Autodesk Fusion 360 part; units mm, degrees
(part 2 of 5)
  line L948 (107.395, 88.0223) -> (106.594, 88.0223)
  line L949 (102.344, 88.0223) -> (102.344, 93.8223)
  line L950 (121.394, 96.9215) -> (121.394, 97.9219)
  line L951 (50.2447, 93.8223) -> (50.2447, 88.0223)
  line L952 (107.395, 96.9215) -> (106.594, 96.9215)
  line L953 (68.4939, 93.8223) -> (69.2947, 93.8223)
  line L954 (87.5439, 96.9215) -> (87.5439, 93.8223)
  line L955 (88.3447, 96.9215) -> (87.5439, 96.9215)
  line L956 (35.669, 93.8223) -> (36.4698, 93.8223)
  line L957 (2.6197, 97.9219) -> (2.6197, 96.9215)
  line L958 (2.6197, 96.9215) -> (1.819, 96.9215)
  line L959 (21.6697, 93.8223) -> (21.6697, 88.0223)
  line L960 (50.2447, 97.9219) -> (50.2447, 96.9215)
  line L961 (88.3447, 83.9227) -> (102.344, 83.9227)
  line L962 (2.6197, 93.8223) -> (2.6197, 88.0223)
  line L963 (2.6197, 88.0223) -> (1.819, 88.0223)
  line L964 (2.6197, 83.9227) -> (16.6192, 83.9227)
  line L965 (88.3447, 84.9217) -> (88.3447, 83.9227)
  line L966 (121.394, 84.9217) -> (122.195, 84.9217)
  line L967 (103.145, 93.8223) -> (103.145, 96.9215)
  line L968 (88.3447, 88.0223) -> (87.5439, 88.0223)
  line L969 (102.344, 97.9219) -> (88.3447, 97.9219)
  line L970 (84.0948, 96.9215) -> (83.294, 96.9215)
  line L971 (87.5439, 88.0223) -> (87.5439, 84.9217)
  line L972 (102.344, 96.9215) -> (102.344, 97.9219)
  line L973 (122.195, 96.9215) -> (121.394, 96.9215)
  line L974 (121.394, 88.0223) -> (121.394, 93.8223)
  line L975 (103.145, 84.9217) -> (103.145, 88.0223)
  line L976 (122.195, 84.9217) -> (122.195, 88.0223)
  line L977 (83.294, 96.9215) -> (83.294, 97.9219)
  line L978 (84.0948, 84.9217) -> (84.0948, 88.0223)
  line L979 (87.5439, 84.9217) -> (88.3447, 84.9217)
  line L980 (87.5439, 93.8223) -> (88.3447, 93.8223)
  line L981 (83.294, 83.9227) -> (83.294, 84.9217)
  line L982 (83.294, 88.0223) -> (83.294, 93.8223)
  line L983 (102.344, 83.9227) -> (102.344, 84.9217)
  line L984 (83.294, 93.8223) -> (84.0948, 93.8223)
  line L985 (107.395, 84.9217) -> (107.395, 83.9227)
  line L986 (102.344, 84.9217) -> (103.145, 84.9217)
  line L987 (84.0948, 93.8223) -> (84.0948, 96.9215)
  line L988 (344.719, 12.8598) -> (345.52, 12.8598)
  line L989 (326.47, 16.9595) -> (326.47, 15.9604)
  line L990 (340.469, 16.9595) -> (326.47, 16.9595)
  line L991 (321.419, 7.0597) -> (321.419, 12.8598)
  line L992 (306.619, 12.8598) -> (307.42, 12.8598)
  line L993 (322.22, 12.8598) -> (322.22, 15.9604)
  line L994 (321.419, 16.9595) -> (307.42, 16.9595)
  line L995 (307.42, 7.0597) -> (306.619, 7.0597)
  line L996 (306.619, 7.0597) -> (306.619, 3.9605)
  line L997 (322.22, 3.9605) -> (322.22, 7.0597)
  line L998 (321.419, 12.8598) -> (322.22, 12.8598)
  line L999 (321.419, 15.9604) -> (321.419, 16.9595)
  line L1000 (306.619, 3.9605) -> (307.42, 3.9605)
  line L1001 (322.22, 15.9604) -> (321.419, 15.9604)
  line L1002 (133.587, 17.6237) -> (133.587, 17.0215)
  line L1003 (307.42, 15.9604) -> (306.619, 15.9604)
  line L1004 (307.42, 12.8598) -> (307.42, 7.0597)
  line L1005 (307.42, 3.9605) -> (307.42, 2.96)
  line L1006 (322.22, 7.0597) -> (321.419, 7.0597)
  line L1007 (307.42, 16.9595) -> (307.42, 15.9604)
  line L1008 (306.619, 15.9604) -> (306.619, 12.8598)
  line L1009 (321.419, 2.96) -> (321.419, 3.9605)
  line L1010 (307.42, 2.96) -> (321.419, 2.96)
  line L1011 (321.419, 3.9605) -> (322.22, 3.9605)
  line L1012 (340.469, 15.9604) -> (340.469, 16.9595)
  line L1013 (132.063, 7.9527) -> (132.063, 12.423)
  line L1014 (166.926, 12.423) -> (166.926, 11.8222)
  line L1015 (133.587, 20.7216) -> (132.788, 20.7216)
  line L1016 (185.688, 11.8222) -> (185.688, 12.423)
  line L1017 (133.587, 21.722) -> (133.587, 20.7216)
  line L1018 (185.688, 7.7225) -> (185.688, 8.7216)
  line L1019 (147.588, 8.7216) -> (148.387, 8.7216)
  line L1020 (186.487, 8.7216) -> (186.487, 11.8222)
  line L1021 (133.587, 8.7216) -> (133.587, 7.7225)
  line L1022 (122.276, 6.7524) -> (125.575, 6.7524)
  line L1023 (133.587, 7.7225) -> (147.588, 7.7225)
  line L1024 (132.788, 20.7216) -> (132.788, 17.6237)
  line L1025 (132.788, 17.6237) -> (133.587, 17.6237)
  line L1026 (219.826, 8.7216) -> (219.826, 11.8222)
  line L1027 (205.026, 7.7225) -> (219.025, 7.7225)
  line L1028 (166.125, 8.7216) -> (166.926, 8.7216)
  line L1029 (205.026, 12.423) -> (205.026, 11.8222)
  line L1030 (219.025, 11.8222) -> (219.025, 12.423)
  line L1031 (185.688, 8.7216) -> (186.487, 8.7216)
  line L1032 (166.926, 11.8222) -> (166.125, 11.8222)
  line L1033 (133.587, 11.8222) -> (132.788, 11.8222)
  line L1034 (147.588, 7.7225) -> (147.588, 8.7216)
  line L1035 (219.025, 8.7216) -> (219.826, 8.7216)
  line L1036 (166.926, 8.7216) -> (166.926, 7.7225)
  line L1037 (219.826, 11.8222) -> (219.025, 11.8222)
  line L1038 (148.387, 11.8222) -> (147.588, 11.8222)
  line L1039 (205.026, 21.722) -> (205.026, 20.7216)
  line L1040 (185.688, 17.0215) -> (185.688, 17.6237)
  line L1041 (147.588, 20.7216) -> (147.588, 21.722)
  line L1042 (219.025, 17.0215) -> (219.025, 17.6237)
  line L1043 (132.788, 8.7216) -> (133.587, 8.7216)
  line L1044 (205.026, 8.7216) -> (205.026, 7.7225)
  line L1045 (219.025, 7.7225) -> (219.025, 8.7216)
  line L1046 (133.587, 12.423) -> (133.587, 11.8222)
  line L1047 (196.751, 12.423) -> (196.751, 7.9527)
  line L1048 (132.788, 11.8222) -> (132.788, 8.7216)
  line L1049 (148.387, 8.7216) -> (148.387, 11.8222)
  line L1050 (166.926, 7.7225) -> (185.688, 7.7225)
  line L1051 (203.501, 17.0215) -> (203.501, 19.2517)
  line L1052 (186.487, 11.8222) -> (185.688, 11.8222)
  line L1053 (204.225, 17.6237) -> (205.026, 17.6237)
  line L1054 (202.501, 20.2517) -> (197.751, 20.2517)
  line L1055 (186.487, 20.7216) -> (185.688, 20.7216)
  line L1056 (166.125, 17.6237) -> (166.926, 17.6237)
  line L1057 (204.225, 11.8222) -> (204.225, 8.7216)
  line L1058 (205.026, 11.8222) -> (204.225, 11.8222)
  line L1059 (166.125, 11.8222) -> (166.125, 8.7216)
  line L1060 (219.025, 17.6237) -> (219.826, 17.6237)
  line L1061 (204.225, 8.7216) -> (205.026, 8.7216)
  line L1062 (147.588, 11.8222) -> (147.588, 12.423)
  line L1063 (219.025, 21.722) -> (205.026, 21.722)
  line L1064 (148.387, 20.7216) -> (147.588, 20.7216)
  line L1065 (281.226, 17.6237) -> (281.226, 11.8222)
  line L1066 (281.226, 11.8222) -> (280.425, 11.8222)
  line L1067 (296.026, 8.7216) -> (296.026, 11.8222)
  line L1068 (219.025, 20.7216) -> (219.025, 21.722)
  line L1069 (204.225, 20.7216) -> (204.225, 17.6237)
  line L1070 (280.425, 11.8222) -> (280.425, 8.7216)
  line L1071 (186.487, 17.6237) -> (186.487, 20.7216)
  line L1072 (280.425, 8.7216) -> (281.226, 8.7216)
  line L1073 (281.226, 21.722) -> (281.226, 20.7216)
  line L1074 (166.926, 21.722) -> (166.926, 20.7216)
  line L1075 (205.026, 17.6237) -> (205.026, 17.0215)
  line L1076 (185.688, 21.722) -> (166.926, 21.722)
  line L1077 (185.688, 20.7216) -> (185.688, 21.722)
  line L1078 (185.688, 17.6237) -> (186.487, 17.6237)
  line L1079 (280.425, 17.6237) -> (281.226, 17.6237)
  line L1080 (295.225, 17.6237) -> (296.026, 17.6237)
  line L1081 (281.226, 20.7216) -> (280.425, 20.7216)
  line L1082 (148.387, 17.6237) -> (148.387, 20.7216)
  line L1083 (295.225, 8.7216) -> (296.026, 8.7216)
  line L1084 (295.225, 20.7216) -> (295.225, 21.722)
  line L1085 (154.863, 20.2517) -> (150.112, 20.2517)
  line L1086 (296.026, 17.6237) -> (296.026, 20.7216)
  line L1087 (296.026, 11.8222) -> (295.225, 11.8222)
  line L1088 (219.826, 17.6237) -> (219.826, 20.7216)
  line L1089 (238.362, 21.722) -> (238.362, 20.7216)
  line L1090 (281.226, 7.7225) -> (295.225, 7.7225)
  line L1091 (166.926, 20.7216) -> (166.125, 20.7216)
  line L1092 (296.026, 20.7216) -> (295.225, 20.7216)
  line L1093 (147.588, 17.6237) -> (148.387, 17.6237)
  line L1094 (205.026, 20.7216) -> (204.225, 20.7216)
  line L1095 (166.926, 17.6237) -> (166.926, 17.0215)
  line L1096 (295.225, 21.722) -> (281.226, 21.722)
  line L1097 (147.588, 21.722) -> (133.587, 21.722)
  line L1098 (166.125, 20.7216) -> (166.125, 17.6237)
  line L1099 (280.425, 20.7216) -> (280.425, 17.6237)
  line L1100 (281.226, 8.7216) -> (281.226, 7.7225)
  line L1101 (237.563, 20.7216) -> (237.563, 17.6237)
  line L1102 (295.225, 7.7225) -> (295.225, 8.7216)
  line L1103 (147.588, 17.0215) -> (147.588, 17.6237)
  line L1104 (238.362, 20.7216) -> (237.563, 20.7216)
  line L1105 (95.4871, 11.8222) -> (94.6877, 11.8222)
  line L1106 (21.6697, 17.6237) -> (21.6697, 11.8222)
  line L1107 (21.6697, 20.7216) -> (20.869, 20.7216)
  line L1108 (67.4261, 11.8222) -> (66.6253, 11.8222)
  line L1109 (95.4871, 17.6237) -> (95.4871, 11.8222)
  line L1110 (52.626, 21.722) -> (52.626, 20.7216)
  line L1111 (295.225, 11.8222) -> (295.225, 17.6237)
  line L1112 (237.563, 17.6237) -> (238.362, 17.6237)
  line L1113 (238.362, 7.7225) -> (252.361, 7.7225)
  line L1114 (252.361, 7.7225) -> (252.361, 8.7216)
  line L1115 (238.362, 8.7216) -> (238.362, 7.7225)
  line L1116 (20.869, 17.6237) -> (21.6697, 17.6237)
  line L1117 (66.6253, 8.7216) -> (67.4261, 8.7216)
  line L1118 (219.826, 20.7216) -> (219.025, 20.7216)
  line L1119 (237.563, 8.7216) -> (238.362, 8.7216)
  line L1120 (252.361, 11.8222) -> (252.361, 17.6237)
  line L1121 (51.8252, 11.8222) -> (51.8252, 8.7216)
  line L1122 (51.8252, 8.7216) -> (52.626, 8.7216)
  line L1123 (94.6877, 20.7216) -> (94.6877, 17.6237)
  line L1124 (20.869, 20.7216) -> (20.869, 17.6237)
  line L1125 (238.362, 11.8222) -> (237.563, 11.8222)
  line L1126 (20.869, 11.8222) -> (20.869, 8.7216)
  line L1127 (20.869, 8.7216) -> (21.6697, 8.7216)
  line L1128 (253.162, 17.6237) -> (253.162, 20.7216)
  line L1129 (95.4871, 8.7216) -> (95.4871, 7.7225)
  line L1130 (66.6253, 11.8222) -> (66.6253, 17.6237)
  line L1131 (52.626, 17.6237) -> (52.626, 11.8222)
  line L1132 (252.361, 8.7216) -> (253.162, 8.7216)
  line L1133 (21.6697, 11.8222) -> (20.869, 11.8222)
  line L1134 (110.287, 17.6237) -> (110.287, 20.7216)
  line L1135 (52.626, 11.8222) -> (51.8252, 11.8222)
  line L1136 (21.6697, 21.722) -> (21.6697, 20.7216)
  line L1137 (252.361, 21.722) -> (238.362, 21.722)
  line L1138 (252.361, 20.7216) -> (252.361, 21.722)
  line L1139 (51.8252, 17.6237) -> (52.626, 17.6237)
  line L1140 (94.6877, 8.7216) -> (95.4871, 8.7216)
  line L1141 (66.6253, 17.6237) -> (67.4261, 17.6237)
  line L1142 (52.626, 7.7225) -> (66.6253, 7.7225)
  line L1143 (253.162, 20.7216) -> (252.361, 20.7216)
  line L1144 (109.488, 7.7225) -> (109.488, 8.7216)
  line L1145 (67.4261, 20.7216) -> (66.6253, 20.7216)
  line L1146 (95.4871, 21.722) -> (95.4871, 20.7216)
  line L1147 (110.287, 11.8222) -> (109.488, 11.8222)
  line L1148 (109.488, 11.8222) -> (109.488, 17.6237)
  line L1149 (252.361, 17.6237) -> (253.162, 17.6237)
  line L1150 (253.162, 8.7216) -> (253.162, 11.8222)
  line L1151 (109.488, 21.722) -> (95.4871, 21.722)
  line L1152 (52.626, 8.7216) -> (52.626, 7.7225)
  line L1153 (95.4871, 20.7216) -> (94.6877, 20.7216)
  line L1154 (94.6877, 17.6237) -> (95.4871, 17.6237)
  line L1155 (253.162, 11.8222) -> (252.361, 11.8222)
  line L1156 (109.488, 8.7216) -> (110.287, 8.7216)
  line L1157 (206.606, 27.7716) -> (207.407, 27.7716)
  line L1158 (202.357, 36.6737) -> (203.156, 36.6737)
  line L1159 (149.456, 30.8722) -> (149.456, 27.7716)
  line L1160 (164.257, 30.8722) -> (164.257, 36.6737)
  line L1161 (221.407, 26.7725) -> (221.407, 27.7716)
  line L1162 (187.556, 39.7715) -> (187.556, 36.6737)
  line L1163 (150.257, 26.7725) -> (164.257, 26.7725)
  line L1164 (187.556, 27.7716) -> (188.357, 27.7716)
  line L1165 (202.357, 27.7716) -> (203.156, 27.7716)
  line L1166 (222.206, 30.8722) -> (221.407, 30.8722)
  line L1167 (168.506, 30.8722) -> (168.506, 27.7716)
  line L1168 (168.506, 27.7716) -> (169.307, 27.7716)
  line L1169 (183.307, 26.7725) -> (183.307, 27.7716)
  line L1170 (184.106, 39.7715) -> (183.307, 39.7715)
  line L1171 (203.156, 39.7715) -> (202.357, 39.7715)
  line L1172 (183.307, 39.7715) -> (183.307, 40.7719)
  line L1173 (188.357, 26.7725) -> (202.357, 26.7725)
  line L1174 (165.056, 36.6737) -> (165.056, 39.7715)
  line L1175 (221.407, 36.6737) -> (222.206, 36.6737)
  line L1176 (169.307, 27.7716) -> (169.307, 26.7725)
  line L1177 (165.056, 30.8722) -> (164.257, 30.8722)
  line L1178 (169.307, 40.7719) -> (169.307, 39.7715)
  line L1179 (169.307, 30.8722) -> (168.506, 30.8722)
  line L1180 (203.156, 36.6737) -> (203.156, 39.7715)
  line L1181 (150.257, 36.6737) -> (150.257, 30.8722)
  line L1182 (221.407, 30.8722) -> (221.407, 36.6737)
  line L1183 (150.257, 27.7716) -> (150.257, 26.7725)
  line L1184 (169.307, 39.7715) -> (168.506, 39.7715)
  line L1185 (184.106, 27.7716) -> (184.106, 30.8722)
  line L1186 (203.156, 30.8722) -> (202.357, 30.8722)
  line L1187 (168.506, 39.7715) -> (168.506, 36.6737)
  line L1188 (149.456, 27.7716) -> (150.257, 27.7716)
  line L1189 (150.257, 30.8722) -> (149.456, 30.8722)
  line L1190 (164.257, 36.6737) -> (165.056, 36.6737)
  line L1191 (188.357, 39.7715) -> (187.556, 39.7715)
  line L1192 (188.357, 36.6737) -> (188.357, 30.8722)
  line L1193 (202.357, 26.7725) -> (202.357, 27.7716)
  line L1194 (203.156, 27.7716) -> (203.156, 30.8722)
  line L1195 (207.407, 26.7725) -> (221.407, 26.7725)
  line L1196 (221.407, 27.7716) -> (222.206, 27.7716)
  line L1197 (164.257, 27.7716) -> (165.056, 27.7716)
  line L1198 (169.307, 26.7725) -> (183.307, 26.7725)
  line L1199 (202.357, 30.8722) -> (202.357, 36.6737)
  line L1200 (202.357, 39.7715) -> (202.357, 40.7719)
  line L1201 (222.206, 27.7716) -> (222.206, 30.8722)
  line L1202 (150.257, 40.7719) -> (150.257, 39.7715)
  line L1203 (183.307, 36.6737) -> (184.106, 36.6737)
  line L1204 (184.106, 36.6737) -> (184.106, 39.7715)
  line L1205 (183.307, 30.8722) -> (183.307, 36.6737)
  line L1206 (169.307, 36.6737) -> (169.307, 30.8722)
  line L1207 (164.257, 26.7725) -> (164.257, 27.7716)
  line L1208 (165.056, 27.7716) -> (165.056, 30.8722)
  line L1209 (202.357, 40.7719) -> (188.357, 40.7719)
  line L1210 (360.32, 12.8598) -> (360.32, 15.9604)
  line L1211 (326.47, 15.9604) -> (325.669, 15.9604)
  line L1212 (345.52, 16.9595) -> (345.52, 15.9604)
  line L1213 (344.719, 3.9605) -> (345.52, 3.9605)
  line L1214 (325.669, 15.9604) -> (325.669, 12.8598)
  line L1215 (341.27, 15.9604) -> (340.469, 15.9604)
  line L1216 (183.307, 27.7716) -> (184.106, 27.7716)
  line L1217 (188.357, 30.8722) -> (187.556, 30.8722)
  line L1218 (150.257, 39.7715) -> (149.456, 39.7715)
  line L1219 (183.307, 40.7719) -> (169.307, 40.7719)
  line L1220 (340.469, 2.96) -> (340.469, 3.9605)
  line L1221 (326.47, 3.9605) -> (326.47, 2.96)
  line L1222 (345.52, 15.9604) -> (344.719, 15.9604)
  line L1223 (359.519, 12.8598) -> (360.32, 12.8598)
  line L1224 (341.27, 3.9605) -> (341.27, 7.0597)
  line L1225 (345.52, 7.0597) -> (344.719, 7.0597)
  line L1226 (359.519, 2.96) -> (359.519, 3.9605)
  line L1227 (360.32, 7.0597) -> (359.519, 7.0597)
  line L1228 (345.52, 3.9605) -> (345.52, 2.96)
  line L1229 (359.519, 16.9595) -> (345.52, 16.9595)
  line L1230 (325.669, 3.9605) -> (326.47, 3.9605)
  line L1231 (168.506, 36.6737) -> (169.307, 36.6737)
  line L1232 (341.27, 12.8598) -> (341.27, 15.9604)
  line L1233 (344.719, 7.0597) -> (344.719, 3.9605)
  line L1234 (360.32, 15.9604) -> (359.519, 15.9604)
  line L1235 (344.719, 15.9604) -> (344.719, 12.8598)
  line L1236 (221.407, 39.7715) -> (221.407, 40.7719)
  line L1237 (149.456, 36.6737) -> (150.257, 36.6737)
  line L1238 (345.52, 2.96) -> (359.519, 2.96)
  line L1239 (326.47, 12.8598) -> (326.47, 7.0597)
  line L1240 (187.556, 30.8722) -> (187.556, 27.7716)
  line L1241 (187.556, 36.6737) -> (188.357, 36.6737)
  line L1242 (149.456, 39.7715) -> (149.456, 36.6737)
  line L1243 (341.27, 7.0597) -> (340.469, 7.0597)
  line L1244 (359.519, 3.9605) -> (360.32, 3.9605)
  line L1245 (359.519, 15.9604) -> (359.519, 16.9595)
  line L1246 (359.519, 7.0597) -> (359.519, 12.8598)
  line L1247 (222.206, 39.7715) -> (221.407, 39.7715)
  line L1248 (184.106, 30.8722) -> (183.307, 30.8722)
  line L1249 (222.206, 36.6737) -> (222.206, 39.7715)
  line L1250 (326.47, 2.96) -> (340.469, 2.96)
  line L1251 (340.469, 3.9605) -> (341.27, 3.9605)
  line L1252 (340.469, 7.0597) -> (340.469, 12.8598)
  line L1253 (340.469, 12.8598) -> (341.27, 12.8598)
  line L1254 (360.32, 3.9605) -> (360.32, 7.0597)
  line L1255 (188.357, 27.7716) -> (188.357, 26.7725)
  line L1256 (325.669, 12.8598) -> (326.47, 12.8598)
  line L1257 (325.669, 7.0597) -> (325.669, 3.9605)
  line L1258 (207.407, 27.7716) -> (207.407, 26.7725)
  line L1259 (345.52, 12.8598) -> (345.52, 7.0597)
  line L1260 (221.407, 40.7719) -> (207.407, 40.7719)
  line L1261 (326.47, 7.0597) -> (325.669, 7.0597)
  line L1262 (188.357, 40.7719) -> (188.357, 39.7715)
  line L1263 (135.169, 74.7723) -> (135.97, 74.7723)
  line L1264 (135.97, 64.8727) -> (149.969, 64.8727)
  line L1265 (97.8697, 77.8715) -> (97.0689, 77.8715)
  line L1266 (169.019, 78.8719) -> (155.02, 78.8719)
  line L1267 (149.969, 65.8717) -> (150.77, 65.8717)
  line L1268 (97.0689, 77.8715) -> (97.0689, 74.7723)
  line L1269 (131.72, 65.8717) -> (131.72, 68.9723)
  line L1270 (116.92, 77.8715) -> (116.119, 77.8715)
  line L1271 (135.97, 68.9723) -> (135.169, 68.9723)
  line L1272 (116.92, 64.8727) -> (130.919, 64.8727)
  line L1273 (130.919, 77.8715) -> (130.919, 78.8719)
  line L1274 (116.119, 68.9723) -> (116.119, 65.8717)
  line L1275 (150.77, 74.7723) -> (150.77, 77.8715)
  line L1276 (169.019, 74.7723) -> (169.82, 74.7723)
  line L1277 (169.019, 64.8727) -> (169.019, 65.8717)
  line L1278 (131.72, 74.7723) -> (131.72, 77.8715)
  line L1279 (155.02, 68.9723) -> (154.219, 68.9723)
  line L1280 (130.919, 74.7723) -> (131.72, 74.7723)
  line L1281 (169.82, 74.7723) -> (169.82, 77.8715)
  line L1282 (149.969, 74.7723) -> (150.77, 74.7723)
  line L1283 (135.169, 77.8715) -> (135.169, 74.7723)
  line L1284 (154.219, 68.9723) -> (154.219, 65.8717)
  line L1285 (116.119, 65.8717) -> (116.92, 65.8717)
  line L1286 (131.72, 77.8715) -> (130.919, 77.8715)
  line L1287 (135.169, 68.9723) -> (135.169, 65.8717)
  line L1288 (150.77, 77.8715) -> (149.969, 77.8715)
  line L1289 (130.919, 65.8717) -> (131.72, 65.8717)
  line L1290 (135.97, 74.7723) -> (135.97, 68.9723)
  line L1291 (169.82, 68.9723) -> (169.019, 68.9723)
  line L1292 (116.92, 74.7723) -> (116.92, 68.9723)
  line L1293 (97.8697, 78.8719) -> (97.8697, 77.8715)
  line L1294 (97.0689, 74.7723) -> (97.8697, 74.7723)
  line L1295 (112.67, 74.7723) -> (112.67, 77.8715)
  line L1296 (130.919, 78.8719) -> (116.92, 78.8719)
  line L1297 (92.819, 78.8719) -> (78.8197, 78.8719)
  line L1298 (69.8059, 65.8717) -> (69.8059, 68.9723)
  line L1299 (54.2064, 65.8717) -> (55.0072, 65.8717)
  line L1300 (78.8197, 65.8717) -> (78.8197, 64.8727)
  line L1301 (55.0072, 64.8727) -> (69.0065, 64.8727)
  line L1302 (69.8059, 74.7723) -> (69.8059, 77.8715)
  line L1303 (78.8197, 68.9723) -> (78.0189, 68.9723)
  line L1304 (131.72, 68.9723) -> (130.919, 68.9723)
  line L1305 (93.6198, 77.8715) -> (92.819, 77.8715)
  line L1306 (130.919, 68.9723) -> (130.919, 74.7723)
  line L1307 (69.0065, 77.8715) -> (69.0065, 78.8719)
  line L1308 (78.0189, 65.8717) -> (78.8197, 65.8717)
  line L1309 (92.819, 65.8717) -> (93.6198, 65.8717)
  line L1310 (112.67, 65.8717) -> (112.67, 68.9723)
  line L1311 (69.0065, 64.8727) -> (69.0065, 65.8717)
  line L1312 (69.8059, 77.8715) -> (69.0065, 77.8715)
  line L1313 (69.0065, 78.8719) -> (55.0072, 78.8719)
  line L1314 (21.6697, 78.8719) -> (21.6697, 77.8715)
  line L1315 (135.97, 78.8719) -> (135.97, 77.8715)
  line L1316 (21.6697, 77.8715) -> (20.869, 77.8715)
  line L1317 (54.2064, 68.9723) -> (54.2064, 65.8717)
  line L1318 (111.869, 74.7723) -> (112.67, 74.7723)
  line L1319 (21.6697, 74.7723) -> (21.6697, 68.9723)
  line L1320 (69.0065, 74.7723) -> (69.8059, 74.7723)
  line L1321 (20.869, 77.8715) -> (20.869, 74.7723)
  line L1322 (111.869, 78.8719) -> (97.8697, 78.8719)
  line L1323 (20.869, 74.7723) -> (21.6697, 74.7723)
  line L1324 (54.2064, 77.8715) -> (54.2064, 74.7723)
  line L1325 (78.8197, 64.8727) -> (92.819, 64.8727)
  line L1326 (78.0189, 74.7723) -> (78.8197, 74.7723)
  line L1327 (97.8697, 64.8727) -> (111.869, 64.8727)
  line L1328 (78.8197, 74.7723) -> (78.8197, 68.9723)
  line L1329 (93.6198, 74.7723) -> (93.6198, 77.8715)
  line L1330 (69.8059, 68.9723) -> (69.0065, 68.9723)
  line L1331 (69.0065, 68.9723) -> (69.0065, 74.7723)
  line L1332 (78.0189, 77.8715) -> (78.0189, 74.7723)
  line L1333 (21.6697, 64.8727) -> (35.669, 64.8727)
  line L1334 (20.869, 68.9723) -> (20.869, 65.8717)
  line L1335 (92.819, 68.9723) -> (92.819, 74.7723)
  line L1336 (55.0072, 74.7723) -> (55.0072, 68.9723)
  line L1337 (111.869, 68.9723) -> (111.869, 74.7723)
  line L1338 (36.4698, 65.8717) -> (36.4698, 68.9723)
  line L1339 (93.6198, 65.8717) -> (93.6198, 68.9723)
  line L1340 (78.0189, 68.9723) -> (78.0189, 65.8717)
  line L1341 (92.819, 77.8715) -> (92.819, 78.8719)
  line L1342 (112.67, 68.9723) -> (111.869, 68.9723)
  line L1343 (35.669, 65.8717) -> (36.4698, 65.8717)
  line L1344 (92.819, 74.7723) -> (93.6198, 74.7723)
  line L1345 (21.6697, 65.8717) -> (21.6697, 64.8727)
  line L1346 (20.869, 65.8717) -> (21.6697, 65.8717)
  line L1347 (55.0072, 65.8717) -> (55.0072, 64.8727)
  line L1348 (69.0065, 65.8717) -> (69.8059, 65.8717)
  line L1349 (55.0072, 68.9723) -> (54.2064, 68.9723)
  line L1350 (35.669, 64.8727) -> (35.669, 65.8717)
  line L1351 (92.819, 64.8727) -> (92.819, 65.8717)
  line L1352 (21.6697, 68.9723) -> (20.869, 68.9723)
  line L1353 (78.8197, 77.8715) -> (78.0189, 77.8715)
  line L1354 (93.6198, 68.9723) -> (92.819, 68.9723)
  line L1355 (78.8197, 78.8719) -> (78.8197, 77.8715)
  line L1356 (112.67, 77.8715) -> (111.869, 77.8715)
  line L1357 (55.0072, 77.8715) -> (54.2064, 77.8715)
  line L1358 (54.2064, 74.7723) -> (55.0072, 74.7723)
  line L1359 (297.094, 96.9215) -> (297.094, 93.8223)
  line L1360 (304.169, 82.9525) -> (304.169, 83.9227)
  line L1361 (331.745, 88.0223) -> (330.944, 88.0223)
  line L1362 (16.6192, 78.8719) -> (2.6196, 78.8719)
  line L1363 (111.869, 77.8715) -> (111.869, 78.8719)
  line L1364 (16.6192, 64.8727) -> (16.6192, 65.8717)
  line L1365 (35.669, 77.8715) -> (35.669, 78.8719)
  line L1366 (2.6197, 74.7723) -> (2.6197, 68.9723)
  line L1367 (111.869, 64.8727) -> (111.869, 65.8717)
  line L1368 (35.669, 68.9723) -> (35.669, 74.7723)
  line L1369 (17.4198, 65.8717) -> (17.4198, 68.9723)
  line L1370 (331.745, 93.8223) -> (331.745, 96.9215)
  line L1371 (297.094, 93.8223) -> (297.895, 93.8223)
  line L1372 (330.944, 97.9219) -> (297.895, 97.9219)
  line L1373 (349.481, 96.9215) -> (349.481, 93.8223)
  line L1374 (55.0072, 78.8719) -> (55.0072, 77.8715)
  line L1375 (324.67, 82.9525) -> (327.969, 82.9525)
  line L1376 (297.895, 84.9217) -> (297.895, 83.9227)
  line L1377 (111.869, 65.8717) -> (112.67, 65.8717)
  line L1378 (350.282, 93.8223) -> (350.282, 88.0223)
  line L1379 (297.895, 97.9219) -> (297.895, 96.9215)
  line L1380 (2.6197, 77.8715) -> (1.819, 77.8715)
  line L1381 (36.4698, 68.9723) -> (35.669, 68.9723)
  line L1382 (330.944, 93.8223) -> (331.745, 93.8223)
  line L1383 (297.895, 88.0223) -> (297.094, 88.0223)
  line L1384 (297.895, 83.9227) -> (300.87, 83.9227)
  line L1385 (327.969, 82.9525) -> (327.969, 83.9227)
  line L1386 (327.969, 83.9227) -> (330.944, 83.9227)
  line L1387 (300.87, 82.9525) -> (304.169, 82.9525)
  line L1388 (2.6197, 78.8719) -> (2.6197, 77.8715)
  line L1389 (304.169, 83.9227) -> (324.67, 83.9227)
  line L1390 (278.044, 84.9217) -> (278.845, 84.9217)
  line L1391 (274.595, 88.0223) -> (273.794, 88.0223)
  line L1392 (16.6192, 65.8717) -> (17.4198, 65.8717)
  line L1393 (2.6197, 65.8717) -> (2.6197, 64.8727)
  line L1394 (17.4198, 74.7723) -> (17.4198, 77.8715)
  line L1395 (17.4198, 68.9723) -> (16.6192, 68.9723)
  line L1396 (349.481, 93.8223) -> (350.282, 93.8223)
  line L1397 (1.819, 74.7723) -> (2.6197, 74.7723)
  line L1398 (17.4198, 77.8715) -> (16.6192, 77.8715)
  line L1399 (278.044, 88.0223) -> (278.044, 84.9217)
  line L1400 (258.994, 84.9217) -> (259.795, 84.9217)
  line L1401 (297.094, 88.0223) -> (297.094, 84.9217)
  line L1402 (1.819, 68.9723) -> (1.819, 65.8717)
  line L1403 (1.819, 77.8715) -> (1.819, 74.7723)
  line L1404 (1.819, 65.8717) -> (2.6197, 65.8717)
  line L1405 (300.87, 83.9227) -> (300.87, 82.9525)
  line L1406 (330.944, 84.9217) -> (331.745, 84.9217)
  line L1407 (297.094, 84.9217) -> (297.895, 84.9217)
  line L1408 (35.669, 78.8719) -> (21.6697, 78.8719)
  line L1409 (16.6192, 77.8715) -> (16.6192, 78.8719)
  line L1410 (297.895, 96.9215) -> (297.094, 96.9215)
  line L1411 (35.669, 74.7723) -> (36.4698, 74.7723)
  line L1412 (16.6192, 74.7723) -> (17.4198, 74.7723)
  line L1413 (331.745, 96.9215) -> (330.944, 96.9215)
  line L1414 (331.745, 84.9217) -> (331.745, 88.0223)
  line L1415 (2.6197, 64.8727) -> (16.6192, 64.8727)
  line L1416 (330.944, 96.9215) -> (330.944, 97.9219)
  line L1417 (16.6192, 68.9723) -> (16.6192, 74.7723)
  line L1418 (350.282, 88.0223) -> (349.481, 88.0223)
  line L1419 (297.895, 93.8223) -> (297.895, 88.0223)
  line L1420 (36.4698, 74.7723) -> (36.4698, 77.8715)
  line L1421 (330.944, 88.0223) -> (330.944, 93.8223)
  line L1422 (349.481, 84.9217) -> (350.282, 84.9217)
  line L1423 (350.282, 84.9217) -> (350.282, 83.9227)
  line L1424 (324.67, 83.9227) -> (324.67, 82.9525)
  line L1425 (350.282, 97.9219) -> (350.282, 96.9215)
  line L1426 (350.282, 96.9215) -> (349.481, 96.9215)
  line L1427 (292.844, 93.8223) -> (293.645, 93.8223)
  line L1428 (278.845, 97.9219) -> (278.845, 96.9215)
  line L1429 (364.282, 93.8223) -> (365.083, 93.8223)
  line L1430 (292.844, 83.9227) -> (292.844, 84.9217)
  line L1431 (273.794, 84.9217) -> (274.595, 84.9217)
  line L1432 (365.083, 96.9215) -> (364.282, 96.9215)
  line L1433 (36.4698, 77.8715) -> (35.669, 77.8715)
  line L1434 (330.944, 83.9227) -> (330.944, 84.9217)
  line L1435 (364.282, 96.9215) -> (364.282, 97.9219)
  line L1436 (2.6197, 68.9723) -> (1.819, 68.9723)
  line L1437 (349.481, 88.0223) -> (349.481, 84.9217)
  line L1438 (258.994, 88.0223) -> (258.994, 84.9217)
  line L1439 (364.282, 88.0223) -> (364.282, 93.8223)
  line L1440 (240.745, 97.9219) -> (240.745, 96.9215)
  line L1441 (240.745, 96.9215) -> (239.944, 96.9215)
  line L1442 (239.944, 93.8223) -> (240.745, 93.8223)
  line L1443 (240.745, 93.8223) -> (240.745, 88.0223)
  line L1444 (240.745, 88.0223) -> (239.944, 88.0223)
  line L1445 (278.044, 93.8223) -> (278.845, 93.8223)
  line L1446 (274.595, 93.8223) -> (274.595, 96.9215)
  line L1447 (273.794, 93.8223) -> (274.595, 93.8223)
  line L1448 (239.944, 84.9217) -> (240.745, 84.9217)
  line L1449 (240.745, 83.9227) -> (254.744, 83.9227)
  line L1450 (254.744, 83.9227) -> (254.744, 84.9217)
  line L1451 (365.083, 88.0223) -> (364.282, 88.0223)
  line L1452 (273.794, 83.9227) -> (273.794, 84.9217)
  line L1453 (364.282, 97.9219) -> (350.282, 97.9219)
  line L1454 (278.845, 96.9215) -> (278.044, 96.9215)
  line L1455 (365.083, 93.8223) -> (365.083, 96.9215)
  line L1456 (240.745, 84.9217) -> (240.745, 83.9227)
  line L1457 (255.545, 84.9217) -> (255.545, 88.0223)
  line L1458 (278.845, 88.0223) -> (278.044, 88.0223)
  line L1459 (292.844, 97.9219) -> (278.845, 97.9219)
  line L1460 (254.744, 84.9217) -> (255.545, 84.9217)
  line L1461 (274.595, 96.9215) -> (273.794, 96.9215)
  line L1462 (292.844, 96.9215) -> (292.844, 97.9219)
  line L1463 (259.795, 88.0223) -> (258.994, 88.0223)
  line L1464 (239.944, 96.9215) -> (239.944, 93.8223)
  line L1465 (239.944, 88.0223) -> (239.944, 84.9217)
  line L1466 (278.845, 93.8223) -> (278.845, 88.0223)
  line L1467 (273.794, 88.0223) -> (273.794, 93.8223)
  line L1468 (292.844, 84.9217) -> (293.645, 84.9217)
  line L1469 (273.794, 97.9219) -> (259.795, 97.9219)
  line L1470 (259.795, 93.8223) -> (259.795, 88.0223)
  line L1471 (292.844, 88.0223) -> (292.844, 93.8223)
  line L1472 (259.795, 96.9215) -> (258.994, 96.9215)
  line L1473 (293.645, 88.0223) -> (292.844, 88.0223)
  line L1474 (364.282, 84.9217) -> (365.083, 84.9217)
  line L1475 (293.645, 96.9215) -> (292.844, 96.9215)
  line L1476 (278.845, 84.9217) -> (278.845, 83.9227)
  line L1477 (235.694, 97.9219) -> (221.695, 97.9219)
  line L1478 (202.645, 97.9219) -> (202.645, 96.9215)
  line L1479 (183.595, 96.9215) -> (182.794, 96.9215)
  line L1480 (182.794, 96.9215) -> (182.794, 93.8223)
  line L1481 (183.595, 93.8223) -> (183.595, 88.0223)
  line L1482 (201.844, 93.8223) -> (202.645, 93.8223)
  line L1483 (235.694, 84.9217) -> (236.495, 84.9217)
  line L1484 (350.282, 83.9227) -> (364.282, 83.9227)
  line L1485 (182.794, 88.0223) -> (182.794, 84.9217)
  line L1486 (198.395, 84.9217) -> (198.395, 88.0223)
  line L1487 (197.594, 88.0223) -> (197.594, 93.8223)
  line L1488 (273.794, 96.9215) -> (273.794, 97.9219)
  line L1489 (197.594, 84.9217) -> (198.395, 84.9217)
  line L1490 (182.794, 84.9217) -> (183.595, 84.9217)
  line L1491 (258.994, 93.8223) -> (259.795, 93.8223)
  line L1492 (293.645, 84.9217) -> (293.645, 88.0223)
  line L1493 (236.495, 88.0223) -> (235.694, 88.0223)
  line L1494 (216.644, 96.9215) -> (216.644, 97.9219)
  line L1495 (183.595, 83.9227) -> (197.594, 83.9227)
  line L1496 (197.594, 83.9227) -> (197.594, 84.9217)
  line L1497 (255.545, 96.9215) -> (254.744, 96.9215)
  line L1498 (236.495, 96.9215) -> (235.694, 96.9215)
  line L1499 (216.644, 84.9217) -> (217.445, 84.9217)
  line L1500 (216.644, 97.9219) -> (202.645, 97.9219)
  line L1501 (259.795, 97.9219) -> (259.795, 96.9215)
  line L1502 (183.595, 84.9217) -> (183.595, 83.9227)
  line L1503 (202.645, 83.9227) -> (216.644, 83.9227)
  line L1504 (198.395, 88.0223) -> (197.594, 88.0223)
  line L1505 (259.795, 84.9217) -> (259.795, 83.9227)
  line L1506 (221.695, 96.9215) -> (220.894, 96.9215)
  line L1507 (220.894, 93.8223) -> (221.695, 93.8223)
  line L1508 (278.845, 83.9227) -> (292.844, 83.9227)
  line L1509 (293.645, 93.8223) -> (293.645, 96.9215)
  line L1510 (236.495, 84.9217) -> (236.495, 88.0223)
  line L1511 (254.744, 96.9215) -> (254.744, 97.9219)
  line L1512 (255.545, 93.8223) -> (255.545, 96.9215)
  line L1513 (259.795, 83.9227) -> (273.794, 83.9227)
  line L1514 (365.083, 84.9217) -> (365.083, 88.0223)
  line L1515 (274.595, 84.9217) -> (274.595, 88.0223)
  line L1516 (364.282, 83.9227) -> (364.282, 84.9217)
  line L1517 (278.044, 96.9215) -> (278.044, 93.8223)
  line L1518 (258.994, 96.9215) -> (258.994, 93.8223)
  line L1519 (201.844, 84.9217) -> (202.645, 84.9217)
  line L1520 (217.445, 93.8223) -> (217.445, 96.9215)
  line L1521 (221.695, 84.9217) -> (221.695, 83.9227)
  line L1522 (220.894, 96.9215) -> (220.894, 93.8223)
  line L1523 (202.645, 84.9217) -> (202.645, 83.9227)
  line L1524 (235.694, 83.9227) -> (235.694, 84.9217)
  line L1525 (254.744, 93.8223) -> (255.545, 93.8223)
  line L1526 (221.695, 88.0223) -> (220.894, 88.0223)
  line L1527 (236.495, 93.8223) -> (236.495, 96.9215)
  line L1528 (217.445, 88.0223) -> (216.644, 88.0223)
  line L1529 (254.744, 88.0223) -> (254.744, 93.8223)
  line L1530 (183.595, 88.0223) -> (182.794, 88.0223)
  line L1531 (197.594, 97.9219) -> (183.595, 97.9219)
  line L1532 (164.545, 93.8223) -> (164.545, 88.0223)
  line L1533 (216.644, 88.0223) -> (216.644, 93.8223)
  line L1534 (144.694, 88.0223) -> (144.694, 84.9217)
  line L1535 (255.545, 88.0223) -> (254.744, 88.0223)
  line L1536 (183.595, 97.9219) -> (183.595, 96.9215)
  line L1537 (235.694, 96.9215) -> (235.694, 97.9219)
  line L1538 (197.594, 93.8223) -> (198.395, 93.8223)
  line L1539 (235.694, 88.0223) -> (235.694, 93.8223)
  line L1540 (220.894, 88.0223) -> (220.894, 84.9217)
  line L1541 (216.644, 83.9227) -> (216.644, 84.9217)
  line L1542 (201.844, 88.0223) -> (201.844, 84.9217)
  line L1543 (221.695, 97.9219) -> (221.695, 96.9215)
  line L1544 (254.744, 97.9219) -> (240.745, 97.9219)
  line L1545 (217.445, 96.9215) -> (216.644, 96.9215)
  line L1546 (202.645, 96.9215) -> (201.844, 96.9215)
  line L1547 (198.395, 93.8223) -> (198.395, 96.9215)
  line L1548 (202.645, 88.0223) -> (201.844, 88.0223)
  line L1549 (221.695, 83.9227) -> (235.694, 83.9227)
  line L1550 (221.695, 93.8223) -> (221.695, 88.0223)
  line L1551 (235.694, 93.8223) -> (236.495, 93.8223)
  line L1552 (220.894, 84.9217) -> (221.695, 84.9217)
  line L1553 (202.645, 93.8223) -> (202.645, 88.0223)
  line L1554 (217.445, 84.9217) -> (217.445, 88.0223)
  line L1555 (216.644, 93.8223) -> (217.445, 93.8223)
  line L1556 (201.844, 96.9215) -> (201.844, 93.8223)
  line L1557 (182.794, 93.8223) -> (183.595, 93.8223)
  line L1558 (173.269, 77.8715) -> (173.269, 74.7723)
  line L1559 (169.019, 77.8715) -> (169.019, 78.8719)
  line L1560 (226.169, 68.9723) -> (226.169, 74.7723)
  line L1561 (226.169, 65.8717) -> (226.97, 65.8717)
  line L1562 (174.07, 77.8715) -> (173.269, 77.8715)
  line L1563 (97.8697, 74.7723) -> (97.8697, 68.9723)
  line L1564 (212.17, 64.8727) -> (226.169, 64.8727)
  line L1565 (207.92, 77.8715) -> (207.119, 77.8715)
  line L1566 (207.119, 78.8719) -> (193.12, 78.8719)
  line L1567 (97.8697, 68.9723) -> (97.0689, 68.9723)
  line L1568 (207.119, 64.8727) -> (207.119, 65.8717)
  line L1569 (211.369, 68.9723) -> (211.369, 65.8717)
  line L1570 (212.17, 65.8717) -> (212.17, 64.8727)
  line L1571 (174.07, 78.8719) -> (174.07, 77.8715)
  line L1572 (149.969, 68.9723) -> (149.969, 74.7723)
  line L1573 (212.17, 77.8715) -> (211.369, 77.8715)
  line L1574 (97.0689, 68.9723) -> (97.0689, 65.8717)
  line L1575 (97.0689, 65.8717) -> (97.8697, 65.8717)
  line L1576 (155.02, 64.8727) -> (169.019, 64.8727)
  line L1577 (135.169, 65.8717) -> (135.97, 65.8717)
  line L1578 (150.77, 68.9723) -> (149.969, 68.9723)
  line L1579 (116.119, 74.7723) -> (116.92, 74.7723)
  line L1580 (149.969, 77.8715) -> (149.969, 78.8719)
  line L1581 (169.82, 65.8717) -> (169.82, 68.9723)
  line L1582 (135.97, 65.8717) -> (135.97, 64.8727)
  line L1583 (169.019, 65.8717) -> (169.82, 65.8717)
  line L1584 (116.119, 77.8715) -> (116.119, 74.7723)
  line L1585 (97.8697, 65.8717) -> (97.8697, 64.8727)
  line L1586 (149.969, 64.8727) -> (149.969, 65.8717)
  line L1587 (169.82, 77.8715) -> (169.019, 77.8715)
  line L1588 (155.02, 65.8717) -> (155.02, 64.8727)
  line L1589 (135.97, 77.8715) -> (135.169, 77.8715)
  line L1590 (154.219, 65.8717) -> (155.02, 65.8717)
  line L1591 (149.969, 78.8719) -> (135.97, 78.8719)
  line L1592 (150.77, 65.8717) -> (150.77, 68.9723)
  line L1593 (169.019, 68.9723) -> (169.019, 74.7723)
  line L1594 (116.92, 78.8719) -> (116.92, 77.8715)
  line L1595 (116.92, 68.9723) -> (116.119, 68.9723)
  line L1596 (116.92, 65.8717) -> (116.92, 64.8727)
  line L1597 (130.919, 64.8727) -> (130.919, 65.8717)
  line L1598 (54.0504, 39.3016) -> (59.6225, 39.3016)
  line L1599 (60.6225, 38.3016) -> (60.6225, 26.8024)
  line L1600 (59.6225, 25.8024) -> (54.0504, 25.8024)
  line L1601 (53.0504, 26.8024) -> (53.0504, 38.3016)
  line L1602 (84.2847, 25.8024) -> (78.676, 25.8024)
  line L1603 (77.676, 26.8024) -> (77.676, 27.0027)
  line L1604 (85.2847, 38.3016) -> (85.2847, 26.8024)
  line L1605 (122.276, 6.7524) -> (120.725, 6.7524)
  line L1606 (154.863, 6.7524) -> (150.112, 6.7524)
  line L1607 (149.112, 7.7524) -> (149.112, 19.2517)
  line L1608 (202.501, 6.7524) -> (197.751, 6.7524)
  line L1609 (227.126, 6.7524) -> (221.551, 6.7524)
  line L1610 (221.551, 20.2517) -> (227.126, 20.2517)
  line L1611 (228.126, 19.2517) -> (228.126, 7.7524)
  line L1612 (285.032, 25.8024) -> (290.607, 25.8024)
  line L1613 (291.607, 26.8024) -> (291.607, 38.3016)
  line L1614 (284.032, 38.3016) -> (284.032, 26.8024)
  line L1615 (315.248, 25.8024) -> (309.657, 25.8024)
  line L1616 (308.657, 26.8024) -> (308.657, 38.3016)
  line L1617 (316.248, 38.3016) -> (316.248, 26.8024)
  line L1618 (296.938, 44.8525) -> (302.513, 44.8525)
  line L1619 (302.513, 58.3516) -> (296.938, 58.3516)
  line L1620 (295.938, 57.3516) -> (295.938, 45.8525)
  line L1621 (327.137, 44.8525) -> (321.562, 44.8525)
  line L1622 (320.562, 45.8525) -> (320.562, 57.3516)
  line L1623 (62.151, 36.0715) -> (62.151, 31.4716)
  line L1624 (78.676, 39.3016) -> (84.2847, 39.3016)
  line L1625 (77.676, 36.0715) -> (77.676, 31.4716)
  line L1626 (76.1503, 36.0715) -> (76.1503, 31.4716)
  line L1627 (119.725, 17.0215) -> (119.725, 19.2517)
  line L1628 (132.063, 19.2517) -> (132.063, 17.0215)
  line L1629 (132.063, 12.423) -> (132.063, 7.7524)
  line L1630 (119.725, 7.7524) -> (119.725, 17.0215)
  line L1631 (120.725, 20.2517) -> (131.063, 20.2517)
  line L1632 (132.063, 17.0215) -> (132.063, 12.423)
  line L1633 (131.063, 6.7524) -> (125.575, 6.7524)
  line L1634 (133.587, 12.423) -> (133.587, 17.0215)
  line L1635 (155.863, 19.2517) -> (155.863, 7.7524)
  line L1636 (166.926, 17.0215) -> (166.926, 12.423)
  line L1637 (147.588, 17.0215) -> (147.588, 12.423)
  line L1638 (205.026, 17.0215) -> (205.026, 12.423)
  line L1639 (185.688, 17.0215) -> (185.688, 12.423)
  line L1640 (203.501, 17.0215) -> (203.501, 7.7524)
  line L1641 (219.025, 17.0215) -> (219.025, 12.423)
  line L1642 (293.132, 36.0715) -> (293.132, 31.4716)
  line L1643 (307.132, 36.0715) -> (307.132, 31.4716)
  line L1644 (303.513, 55.1215) -> (303.513, 45.8525)
  line L1645 (305.037, 55.1215) -> (305.037, 50.5217)
  line L1646 (328.137, 57.3516) -> (328.137, 45.8525)
  line L1647 (319.038, 55.1215) -> (319.038, 50.5217)
  line L1648 (-4.6103, 113.1519) -> (371.512, 113.1519)
  line L1649 (379.512, 105.1519) -> (379.512, -4.27)
  line L1650 (371.512, -12.27) -> (-4.6103, -12.27)
  line L1651 (-12.6103, -4.27) -> (-12.6103, 105.1519)
  arc A0 (-12.6103, -4.27) -> (-4.6103, -12.27) centre (-4.6103, -4.27) ccw
  arc A1 (-4.6103, 113.1519) -> (-12.6103, 105.1519) centre (-4.6103, 105.1519) ccw
  arc A2 (379.512, 105.1519) -> (371.512, 113.1519) centre (371.512, 105.1519) ccw
  arc A3 (371.512, -12.27) -> (379.512, -4.27) centre (371.512, -4.27) ccw
  arc A4 (54.0504, 39.3016) -> (53.0504, 38.3016) centre (54.0504, 38.3016) ccw
  arc A5 (60.6225, 38.3016) -> (59.6225, 39.3016) centre (59.6225, 38.3016) ccw
  arc A6 (53.0504, 26.8024) -> (54.0504, 25.8024) centre (54.0504, 26.8024) ccw
  arc A7 (59.6225, 25.8024) -> (60.6225, 26.8024) centre (59.6225, 26.8024) ccw
  arc A8 (77.676, 26.8024) -> (78.676, 25.8024) centre (78.676, 26.8024) ccw
  arc A9 (84.2847, 25.8024) -> (85.2847, 26.8024) centre (84.2847, 26.8024) ccw
  arc A10 (85.2847, 38.3016) -> (84.2847, 39.3016) centre (84.2847, 38.3016) ccw
  arc A11 (78.676, 39.3016) -> (77.676, 38.3016) centre (78.676, 38.3016) ccw
  arc A12 (120.725, 20.2517) -> (119.725, 19.2517) centre (120.725, 19.2517) ccw
  arc A13 (132.063, 19.2517) -> (131.063, 20.2517) centre (131.063, 19.2517) ccw
  arc A14 (131.063, 6.7524) -> (132.063, 7.7524) centre (131.063, 7.7524) ccw
  arc A15 (119.725, 7.7524) -> (120.725, 6.7524) centre (120.725, 7.7524) ccw
  arc A16 (150.112, 20.2517) -> (149.112, 19.2517) centre (150.112, 19.2517) ccw
  arc A17 (155.863, 19.2517) -> (154.863, 20.2517) centre (154.863, 19.2517) ccw
  arc A18 (154.863, 6.7524) -> (155.863, 7.7524) centre (154.863, 7.7524) ccw
  arc A19 (149.112, 7.7524) -> (150.112, 6.7524) centre (150.112, 7.7524) ccw
  arc A20 (197.751, 20.2517) -> (196.751, 19.2517) centre (197.751, 19.2517) ccw
  arc A21 (203.501, 19.2517) -> (202.501, 20.2517) centre (202.501, 19.2517) ccw
  arc A22 (202.501, 6.7524) -> (203.501, 7.7524) centre (202.501, 7.7524) ccw
  arc A23 (196.751, 7.7524) -> (197.751, 6.7524) centre (197.751, 7.7524) ccw
  line L1652 (196.751, 19.2517) -> (196.751, 12.423)
  arc A24 (221.551, 20.2517) -> (220.551, 19.2517) centre (221.551, 19.2517) ccw
  arc A25 (228.126, 19.2517) -> (227.126, 20.2517) centre (227.126, 19.2517) ccw
  arc A26 (227.126, 6.7524) -> (228.126, 7.7524) centre (227.126, 7.7524) ccw
  arc A27 (220.551, 7.7524) -> (221.551, 6.7524) centre (221.551, 7.7524) ccw
  line L1653 (220.551, 19.2517) -> (220.551, 7.7524)
  arc A28 (284.032, 26.8024) -> (285.032, 25.8024) centre (285.032, 26.8024) ccw
  arc A29 (290.607, 25.8024) -> (291.607, 26.8024) centre (290.607, 26.8024) ccw
  arc A30 (285.032, 39.3016) -> (284.032, 38.3016) centre (285.032, 38.3016) ccw
  arc A31 (291.607, 38.3016) -> (290.607, 39.3016) centre (290.607, 38.3016) ccw
  line L1654 (285.032, 39.3016) -> (290.607, 39.3016)
  arc A32 (309.657, 39.3016) -> (308.657, 38.3016) centre (309.657, 38.3016) ccw
  arc A33 (316.248, 38.3016) -> (315.248, 39.3016) centre (315.248, 38.3016) ccw
  arc A34 (308.657, 26.8024) -> (309.657, 25.8024) centre (309.657, 26.8024) ccw
  arc A35 (315.248, 25.8024) -> (316.248, 26.8024) centre (315.248, 26.8024) ccw
  line L1655 (309.657, 39.3016) -> (315.248, 39.3016)
  arc A36 (295.938, 45.8525) -> (296.938, 44.8525) centre (296.938, 45.8525) ccw
  arc A37 (302.513, 44.8525) -> (303.513, 45.8525) centre (302.513, 45.8525) ccw
  arc A38 (296.938, 58.3516) -> (295.938, 57.3516) centre (296.938, 57.3516) ccw
  arc A39 (303.513, 57.3516) -> (302.513, 58.3516) centre (302.513, 57.3516) ccw
  arc A40 (321.562, 58.3516) -> (320.562, 57.3516) centre (321.562, 57.3516) ccw
  arc A41 (328.137, 57.3516) -> (327.137, 58.3516) centre (327.137, 57.3516) ccw
  arc A42 (327.137, 44.8525) -> (328.137, 45.8525) centre (327.137, 45.8525) ccw
  arc A43 (320.562, 45.8525) -> (321.562, 44.8525) centre (321.562, 45.8525) ccw
  line L1656 (327.137, 58.3516) -> (321.562, 58.3516)
  circle A44 centre (-4.6103, 105.1519) radius 1.55
  circle A45 centre (-4.6103, -4.27) radius 1.55
  circle A46 centre (371.512, -4.27) radius 1.55
  circle A47 centre (371.512, 105.1519) radius 1.55
  point P0 (-4.6103, 105.1519)
  point P1 (-4.6103, -4.27)
  point P2 (371.512, -4.27)
  point P3 (371.512, 105.1519)
  dimension "d1" = 15.23
  dimension "d2" = 15.23
  dimension "d4" = 15.23
  dimension "d5" = 15.23
  dimension "d6" = 8
  dimension "d7" = 1
  dimension "d8" = 1
  dimension "d9" = 1
  dimension "d10" = 1
  dimension "d11" = 1
  dimension "d12" = 1
  dimension "d13" = 1
  dimension "d14" = 1
  dimension "d16" = 3.1
  dimension "d17" = 3.1
  dimension "d18" = 3.1
  dimension "d19" = 3.1
  constraint horizontal L1598
  constraint vertical L1599
  constraint horizontal L1600
  constraint vertical L1601
  constraint horizontal L1602
  constraint vertical L1603
  constraint vertical L1604
  constraint vertical L1628
  constraint horizontal L1605
  constraint horizontal L1606
  constraint vertical L1607
  constraint horizontal L1608
  constraint horizontal L1609
  constraint horizontal L1610
  constraint vertical L1611
  constraint horizontal L1612
  constraint vertical L1613
  constraint vertical L1614
  constraint horizontal L1615
  constraint vertical L1616
  constraint vertical L1617
  constraint horizontal L1618
  constraint horizontal L1619
  constraint vertical L1620
  constraint horizontal L1621
  constraint vertical L1622
  constraint coincident L1599 L256.start
  constraint parallel L259 L1623
  constraint perpendicular L1604 L1624
  constraint perpendicular L1624 L1625
  constraint parallel L312 L1626
  constraint collinear L1628 L1629
  constraint perpendicular L1605 L1630
  constraint perpendicular L1628 L1631
  constraint perpendicular L1629 L1633
  constraint perpendicular L1022 L1634
  constraint perpendicular L1606 L1635
  constraint parallel L1014 L1636
  constraint parallel L1062 L1637
  constraint parallel L1029 L1638
  constraint parallel L1016 L1639
  constraint perpendicular L1608 L1640
  constraint vertical L1641
  constraint parallel L270 L1642
  constraint parallel L265 L1643
  constraint perpendicular L1618 L1644
  constraint parallel L439 L1645
  constraint perpendicular L1621 L1646
  constraint parallel L524 L1647
  constraint horizontal L1648
  constraint vertical L1649
  constraint horizontal L1650
  constraint vertical L1651
  constraint tangent L1650 A0
  constraint tangent L1651 A0
  constraint tangent L1648 A1
  constraint tangent L1651 A1
  constraint equal A0 A1
  constraint tangent L1648 A2
  constraint tangent L1649 A2
  constraint equal A0 A2
  constraint tangent L1649 A3
  constraint tangent L1650 A3
  constraint equal A0 A3
  constraint tangent L1598 A4
  constraint tangent L1601 A4
  constraint tangent L1598 A5
  constraint tangent L1599 A5
  constraint equal A4 A5
  constraint tangent L1600 A6
  constraint tangent L1601 A6
  constraint equal A4 A6
  constraint tangent L1599 A7
  constraint tangent L1600 A7
  constraint equal A4 A7
  constraint tangent L1602 A8
  constraint tangent L1603 A8
  constraint equal A4 A8
  constraint tangent L1602 A9
  constraint tangent L1604 A9
  constraint equal A4 A9
  constraint tangent L1604 A10
  constraint tangent L1624 A10
  constraint equal A4 A10
  constraint tangent L304 A11
  constraint tangent L1624 A11
  constraint equal A4 A11
  constraint tangent L1627 A12
  constraint tangent L1631 A12
  constraint tangent L1628 A13
  constraint tangent L1631 A13
  constraint equal A12 A13
  constraint tangent L1629 A14
  constraint tangent L1633 A14
  constraint equal A12 A14
  constraint tangent L1605 A15
  constraint tangent L1630 A15
  constraint equal A12 A15
  constraint tangent L1085 A16
  constraint equal A12 A16
  constraint tangent L1085 A17
  constraint tangent L1635 A17
  constraint equal A12 A17
  constraint tangent L1606 A18
  constraint tangent L1635 A18
  constraint equal A12 A18
  constraint tangent L1606 A19
  constraint tangent L1607 A19
  constraint equal A12 A19
  constraint tangent L1054 A20
  constraint tangent L1051 A21
  constraint tangent L1054 A21
  constraint equal A20 A21
  constraint tangent L1608 A22
  constraint tangent L1640 A22
  constraint equal A20 A22
  constraint tangent L1608 A23
  constraint equal A20 A23
  constraint tangent A20 L1652
  constraint tangent L1610 A24
  constraint tangent L1610 A25
  constraint tangent L1611 A25
  constraint equal A24 A25
  constraint tangent L1609 A26
  constraint tangent L1611 A26
  constraint equal A24 A26
  constraint tangent L1609 A27
  constraint equal A24 A27
  constraint tangent A27 L1653
  constraint tangent L1612 A28
  constraint tangent L1614 A28
  constraint tangent L1612 A29
  constraint tangent L1613 A29
  constraint equal A28 A29
  constraint tangent L1614 A30
  constraint equal A28 A30
  constraint tangent L233 A31
  constraint equal A28 A31
  constraint tangent A31 L1654
  constraint tangent L1617 A33
  constraint equal A32 A33
  constraint tangent L1615 A34
  constraint tangent L1616 A34
  constraint equal A32 A34
  constraint tangent L1615 A35
  constraint tangent L1617 A35
  constraint equal A32 A35
  constraint tangent A33 L1655
  constraint tangent L1618 A36
  constraint tangent L1620 A36
  constraint tangent L1618 A37
  constraint tangent L1644 A37
  constraint equal A36 A37
  constraint tangent L1619 A38
  constraint tangent L1620 A38
  constraint equal A36 A38
  constraint tangent L456 A39
  constraint tangent L1619 A39
  constraint equal A36 A39
  constraint tangent L1622 A40
  constraint tangent L1646 A41
  constraint equal A40 A41
  constraint tangent L1621 A42
  constraint tangent L1646 A42
  constraint equal A40 A42
  constraint tangent L1621 A43
  constraint tangent L1622 A43
  constraint equal A40 A43
  constraint tangent A40 L1656
  constraint coincident P0 A1.centre
  constraint coincident P1 A0.centre
  constraint coincident P2 A3.centre
  constraint coincident P3 A2.centre
  constraint concentric A1 A44
  constraint concentric A0 A45
  measures "d1" distance of L923 L1648
  measures "d2" distance of L962 L1651
  measures "d4" distance of L1238 L1650
  measures "d5" distance of L317 L1649
  measures "d6" radius of A0
  measures "d7" radius of A4
  measures "d8" radius of A12
  measures "d9" radius of A20
  measures "d10" radius of A24
  measures "d11" radius of A28
  measures "d12" radius of A32
  measures "d13" radius of A36
  measures "d14" radius of A40
  measures "d16" diameter of A44
  measures "d17" diameter of A45
  measures "d18" diameter of A46
  measures "d19" diameter of A47
extrude "Extrude1" add sketch "plate" along normal blind 3 makes body 1